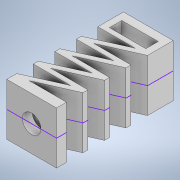
# Autodesk Inventor part: resorte4
Saved by Autodesk Inventor 2021.5 (Build 255421000, 421)
## iProperties
Created: 2024-11-28
Part Number: resorte4
Material: Genérico
Document SubType Name: Modeling
Designer: Joho_
Density: 1 g/cm^3
Appearance: Valor por defecto
Author: Joho_
## iProperties of the stored document _3DPrint.ipt
Created: 2024-11-28
Part Number: _3DPrint
Material: Genérico
Document SubType Name: Modeling
Designer: Joho_
Density: 1 g/cm^3
Appearance: Valor por defecto
Author: Joho_
Autodesk Inventor part; units mm, degrees
ref_plane "YZ Plane" through (0, 0, 0) normal (1, 0, 0) x (0, 1, 0)
ref_plane "XZ Plane" through (0, 0, 0) normal (0, 1, 0) x (-1, 0, 0)
ref_plane "XY Plane" through (0, 0, 0) normal (0, 0, 1) x (1, 0, 0)
sketch "Boceto1" plane through (0, 0, 0) normal (0, 0, 1) x (1, 0, 0)
  circle A0 centre (0, 0) radius 8.9
  line L0 (6.2933, -6.2933) -> (-6.2933, -6.2933)
  line L1 (-6.2933, -6.2933) -> (-6.2933, 6.2933)
  line L2 (-6.2933, 6.2933) -> (6.2933, 6.2933)
  line L3 (6.2933, 6.2933) -> (6.2933, -6.2933)
  circle A1 centre (0, 0) radius 2.25
  dimension "d0" = 17.8
  dimension "d1" = 12.5865
  dimension "d2" = 12.5865
  dimension "d48" = 4.5
  constraints: 8 end point, 2 centre point, 2 coincident, 2 parallel, 1 horizontal, 1 perpendicular
  measures "d0" diameter of A0
  measures "d1" distance of L1.end L2.end
  measures "d2" distance of L0.end L1.end
  measures "d48" diameter of A1
sketch "Boceto2" plane through (0, 0, 0) normal (0, 1, 0) x (-1, 0, 0)
  line L0 (6.2933, 0) -> (-6.2933, 0)
  line L1 (-6.2933, 0) -> (-6.2933, 2)
  line L2 (-6.2933, 2) -> (6.2933, 2)
  line L3 (6.2933, 2) -> (6.2933, 0)
  line L4 (6.2933, 5) -> (-6.2933, 5)
  line L5 (-6.2933, 5) -> (-6.2933, 7)
  line L6 (-6.2933, 7) -> (6.2933, 7)
  line L7 (6.2933, 7) -> (6.2933, 5)
  line L8 (6.2933, 10) -> (-6.2933, 10)
  line L9 (-6.2933, 10) -> (-6.2933, 12)
  line L10 (-6.2933, 12) -> (6.2933, 12)
  line L11 (6.2933, 12) -> (6.2933, 10)
  line L12 (6.2933, 15) -> (-6.2933, 15)
  line L13 (-6.2933, 15) -> (-6.2933, 17)
  line L14 (-6.2933, 17) -> (6.2933, 17)
  line L15 (6.2933, 17) -> (6.2933, 15)
  line L16 (6.2933, 20) -> (-6.2933, 20)
  line L17 (-6.2933, 20) -> (-6.2933, 22)
  line L18 (-6.2933, 22) -> (6.2933, 22)
  line L19 (6.2933, 22) -> (6.2933, 20)
  line L20 (6.2933, 25) -> (-6.2933, 25)
  line L21 (-6.2933, 25) -> (-6.2933, 27)
  line L22 (-6.2933, 27) -> (6.2933, 27)
  line L23 (6.2933, 27) -> (6.2933, 25)
  line L24 (6.2933, 30) -> (-6.2933, 30)
  line L25 (-6.2933, 30) -> (-6.2933, 32)
  line L26 (-6.2933, 32) -> (6.2933, 32)
  line L27 (6.2933, 32) -> (6.2933, 30)
  line L28 (-6.2933, 0) -> (6.2933, 5)
  line L29 (-6.2933, 1.883) -> (6.2933, 6.883)
  line L30 (-6.2933, 6.883) -> (6.2933, 11.883)
  line L31 (-6.2933, 5) -> (6.2933, 10)
  line L32 (-6.2933, 11.883) -> (6.2933, 16.883)
  line L33 (-6.2933, 10) -> (6.2933, 15)
  line L34 (-6.2933, 16.883) -> (6.2933, 21.883)
  line L35 (-6.2933, 15) -> (6.2933, 20)
  line L36 (-6.2933, 21.883) -> (6.2933, 26.883)
  line L37 (-6.2933, 20) -> (6.2933, 25)
  line L38 (-6.2933, 26.883) -> (6.2933, 31.883)
  line L39 (-6.2933, 25) -> (6.2933, 30)
  line L40 (6.2933, 0) -> (4.2933, 0)
  line L41 (4.2933, 0) -> (4.2933, 7)
  line L42 (4.2933, 7) -> (6.2933, 7)
  line L43 (6.2933, 7) -> (6.2933, 0)
  line L44 (-6.2933, 0) -> (-4.2933, 0)
  line L45 (-4.2933, 0) -> (-4.2933, 7)
  line L46 (-4.2933, 7) -> (-6.2933, 7)
  line L47 (-6.2933, 7) -> (-6.2933, 0)
  point P0 (0, 0)
  point P1 (0, 5)
  point P2 (0, 10)
  point P3 (0, 15)
  point P4 (0, 20)
  point P5 (0, 25)
  point P6 (0, 30)
  point P7 (1.5531, 30)
  point P8 (-5.9988, 27)
  point P9 (1.5531, 25)
  point P10 (-5.9988, 22)
  point P11 (1.5531, 20)
  point P12 (-5.9988, 17)
  point P13 (1.5531, 15)
  point P14 (-5.9988, 12)
  point P15 (1.5531, 10)
  point P16 (-5.9988, 7)
  point P17 (1.5531, 5)
  point P18 (-5.9988, 2)
  point P19 (-1.2586, 2)
  point P20 (-1.2587, 7)
  point P21 (-1.2587, 12)
  point P22 (-1.2587, 17)
  point P23 (-1.2586, 22)
  point P24 (-1.2586, 27)
  point P25 (4.2933, 5)
  point P26 (4.2933, 2)
  point P27 (-4.2933, 2)
  point P28 (-4.2933, 5)
  dimension "d11" = 2
  dimension "d12" = 5
  dimension "d13" = 1.75
  dimension "d14" = 5
  dimension "d15" = 2
  dimension "d16" = 2
  constraints: 96 end point, 5 parallel, 4 point on line, 2 horizontal, 2 perpendicular, 2 vertical, 1 coincident, 1 collinear, 83 other
  measures "d11" distance of L0.end L1.end
  measures "d12" distance of point (0, 0) point (0, 5)
  measures "d13" distance between parallel lines of L28 L29
  measures "d14" distance of L29.start L30.start
  measures "d15" distance of L41.end L42.end
  measures "d16" distance of L46.end L45.end
sketch "Boceto3" plane through (0, 0, 0) normal (0, 1, 0) x (-1, 0, 0)
  line L0 (6, 0) -> (-6, 0)
  line L1 (-6, 0) -> (-6, 2)
  line L2 (-4.4, 2) -> (4.4, 2)
  line L3 (6, 2) -> (6, 0)
  line L4 (-6, 0) -> (-4.4, 0)
  line L5 (-4.4, 2) -> (-4.4, 5)
  line L6 (-4.4, 5) -> (-6, 5)
  line L7 (-6, 5) -> (-6, 0)
  line L8 (6, 0) -> (4.4, 0)
  line L9 (4.4, 2) -> (4.4, 5)
  line L10 (4.4, 5) -> (6, 5)
  line L11 (6, 5) -> (6, 0)
  line L12 (6, 5) -> (-6, 5)
  line L13 (-6, 5) -> (-6, 6.2)
  line L14 (-3, 6.2) -> (6, 6.2)
  line L15 (6, 6.2) -> (6, 5)
  line L16 (3, 10.2) -> (6, 10.2)
  line L17 (3, 10.2) -> (-6, 6.2)
  line L18 (6, 10.2) -> (-3, 6.2)
  line L19 (-4.4, 10.2) -> (-6, 10.2)
  line L20 (-6, 10.2) -> (-6, 11.4)
  line L21 (6, 10.2) -> (-6, 10.2)
  line L22 (3, 15.4) -> (-6, 11.4)
  line L23 (-3, 11.4) -> (6, 11.4)
  line L24 (6, 15.4) -> (-3, 11.4)
  line L25 (3, 15.4) -> (6, 15.4)
  line L26 (6, 11.4) -> (6, 10.2)
  line L27 (4.4, 10.2) -> (6, 10.2)
  line L28 (-4.4, 15.4) -> (-6, 15.4)
  line L29 (-6, 15.4) -> (-6, 16.6)
  line L30 (6, 15.4) -> (-6, 15.4)
  line L31 (3, 20.6) -> (-6, 16.6)
  line L32 (-3, 16.6) -> (6, 16.6)
  line L33 (6, 20.6) -> (-3, 16.6)
  line L34 (3, 20.6) -> (6, 20.6)
  line L35 (6, 16.6) -> (6, 15.4)
  line L36 (4.4, 15.4) -> (6, 15.4)
  line L37 (-4.4, 20.6) -> (-6, 20.6)
  line L38 (-6, 20.6) -> (-6, 21.8)
  line L39 (6, 20.6) -> (-6, 20.6)
  line L40 (3, 25.8) -> (-6, 21.8)
  line L41 (-3, 21.8) -> (6, 21.8)
  line L42 (6, 25.8) -> (-3, 21.8)
  line L43 (3, 25.8) -> (6, 25.8)
  line L44 (6, 21.8) -> (6, 20.6)
  line L45 (4.4, 20.6) -> (6, 20.6)
  line L46 (6, 25.8) -> (-6, 25.8)
  line L47 (-6, 25.8) -> (-6, 28.2)
  line L48 (-6, 28.2) -> (6, 28.2)
  line L49 (6, 28.2) -> (6, 25.8)
  point P0 (0, 0)
  dimension "d19" = 12
  dimension "d20" = 2
  dimension "d21" = 1.6
  dimension "d22" = 5
  dimension "d23" = 1.6
  dimension "d24" = 5
  dimension "d25" = 1.2
  dimension "d39" = 5.2
  dimension "d44" = 12
  dimension "d45" = 2.4
  constraints: 100 end point, 11 parallel, 6 horizontal, 5 perpendicular, 1 point on line, 1 vertical, 57 other
  measures "d19" distance of L1.end L3.start
  measures "d20" distance of L0.end L1.end
  measures "d21" distance of L6.end L5.end
  measures "d22" distance of L5.end L4.end
  measures "d23" distance of L9.end L10.end
  measures "d24" distance of L8.end L9.end
  measures "d25" distance of L12.end L13.end
  measures "d39" distance of L5.end L19.start
  measures "d44" distance of L47.end L48.end
  measures "d45" distance of L46.end L47.end
extrude "Extrusión1" add sketch "Boceto1" along normal blind 30 contours L3 L0 L1 L2
extrude "Extrusión2" cut sketch "Boceto3" against normal mid plane 30 contours L0 L1 L7 L6 L5 L2 L9 L10 L11 L3 | L10 L12 L6 L13 L17 L16 L18 L14 L15 | L16 L21 L19 L20 L22 L25 L24 L23 L26 | L25 L30 L28 L29 L31 L34 L33 L32 L35 | L34 L39 L37 L38 L40 L43 L42 L41 L44 | L43 L46 L47 L48 L49 keep common part
sketch "Boceto4" plane through (0, 0, 0) normal (0, 1, 0) x (-1, 0, 0)
  line L0 (-4.4, 2) -> (4.4, 2)
  line L1 (-4.4, 5) -> (-4.4, 2)
  line L2 (4.4, 5) -> (-4.4, 5)
  line L3 (4.4, 2) -> (4.4, 5)
  line L4 (6, 6.2) -> (6, 0)
  line L5 (-3, 6.2) -> (6, 6.2)
  line L6 (6, 10.2) -> (-3, 6.2)
  line L7 (6, 11.4) -> (6, 10.2)
  line L8 (-3, 11.4) -> (6, 11.4)
  line L9 (6, 15.4) -> (-3, 11.4)
  line L10 (6, 16.6) -> (6, 15.4)
  line L11 (-3, 16.6) -> (6, 16.6)
  line L12 (6, 20.6) -> (-3, 16.6)
  line L13 (6, 21.8) -> (6, 20.6)
  line L14 (-3, 21.8) -> (6, 21.8)
  line L15 (6, 25.8) -> (-3, 21.8)
  line L16 (6, 28.2) -> (6, 25.8)
  line L17 (-6, 28.2) -> (6, 28.2)
  line L18 (-6, 25.8) -> (-6, 28.2)
  line L19 (3, 25.8) -> (-6, 25.8)
  line L20 (-6, 21.8) -> (3, 25.8)
  line L21 (-6, 20.6) -> (-6, 21.8)
  line L22 (3, 20.6) -> (-6, 20.6)
  line L23 (-6, 16.6) -> (3, 20.6)
  line L24 (-6, 15.4) -> (-6, 16.6)
  line L25 (3, 15.4) -> (-6, 15.4)
  line L26 (-6, 11.4) -> (3, 15.4)
  line L27 (-6, 10.2) -> (-6, 11.4)
  line L28 (3, 10.2) -> (-6, 10.2)
  line L29 (-6, 6.2) -> (3, 10.2)
  line L30 (-6, 0) -> (-6, 6.2)
  line L31 (-6, 0) -> (6, 0)
  point P0 (0, 0)
  constraints: 64 end point
